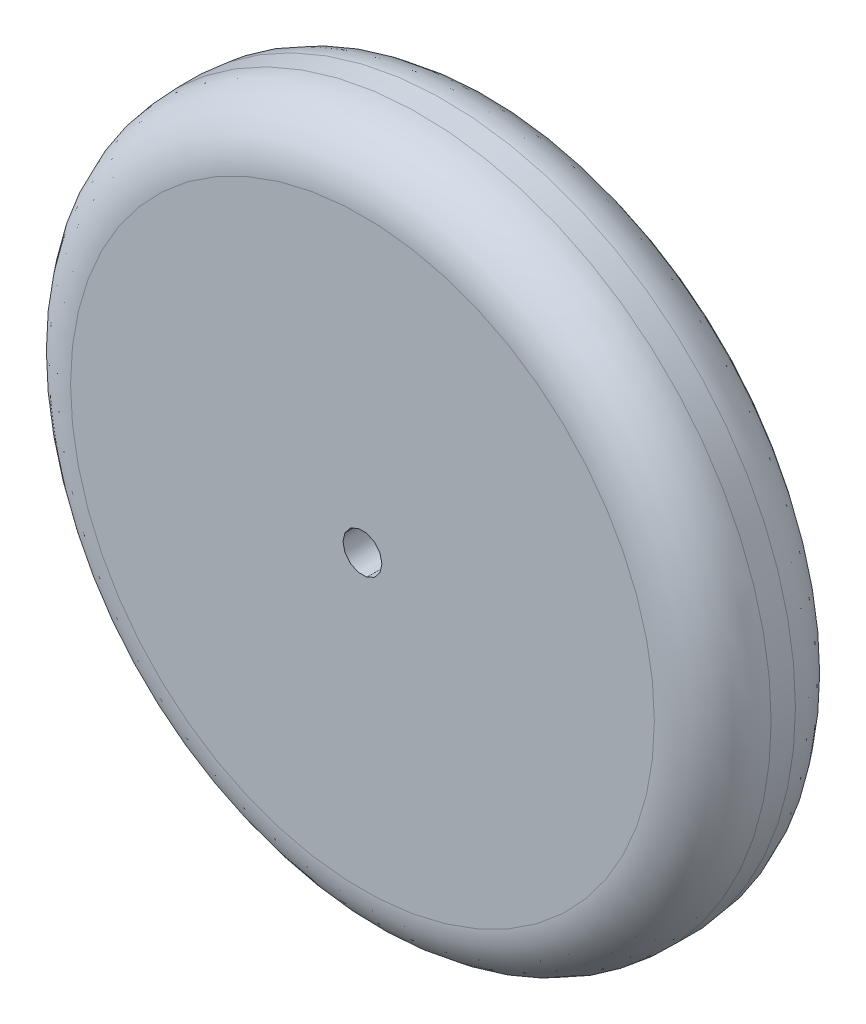
# Autodesk Inventor part: Scooter Wheel
Saved by Autodesk Inventor 2017 (Build 210142000, 142)
## iProperties
Created: 2018-10-18
Part Number: Scooter Wheel
Material: Rubber
Document SubType Name: Modeling
Designer: Administrator
Density: 0.93 g/cm^3
Appearance: Rubber - Black
Author: Administrator
Autodesk Inventor part; units mm, degrees
ref_plane "YZ Plane" through (0, 0, 0) normal (1, 0, 0) x (0, 1, 0)
ref_plane "XZ Plane" through (0, 0, 0) normal (0, 1, 0) x (-1, 0, 0)
ref_plane "XY Plane" through (0, 0, 0) normal (0, 0, 1) x (1, 0, 0)
sketch "Sketch1" plane through (0, 0, 0) normal (0, 0, 1) x (1, 0, 0)
  circle A0 centre (0, 0) radius 4
  circle A1 centre (0, 0) radius 72
  dimension "d0" = 8
  dimension "d1" = 144
  constraints: 2 centre point, 2 coincident
  measures "d0" diameter of A0
  measures "d1" diameter of A1
extrude "Extrusion1" add sketch "Sketch1" along normal blind 29
fillet "Fillet1" radius 12 2 edges at (-72, 0, 29) (-72, 0, 0)
body "Solid1"
